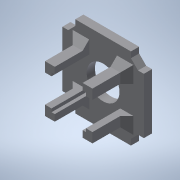
# Autodesk Inventor part: 20_Cube_Insert_Beamsplitter_v3
Saved by Autodesk Inventor 2022 (Build 260153000, 153)
## iProperties
Created: 2019-08-06
Part Number: 20_Cube_Insert_Beamsplitter_v3
Material: Generic
Document SubType Name: Modeling
Designer: marsikovabarbora
Density: 1 g/cm^3
Appearance: Default
Author: marsikovabarbora
Autodesk Inventor part; units mm, degrees
ref_plane "YZ Plane" through (0, 0, 0) normal (1, 0, 0) x (0, 1, 0)
ref_plane "XZ Plane" through (0, 0, 0) normal (0, 1, 0) x (-1, 0, 0)
ref_plane "XY Plane" through (0, 0, 0) normal (0, 0, 1) x (1, 0, 0)
sketch "Sketch1" plane through (0, 0, 0) normal (0, 0, 1) x (1, 0, 0)
  line L0 (-34.86, 0) -> (34.86, 0) construction
  line L1 (0, -34.86) -> (0, 34.86) construction
  line L2 (0, 0) -> (16.9726, 16.9726) construction
  line L3 (0, 0) -> (24.0028, 0) construction
  line L4 (0, 24.9) -> (16.8009, 24.9)
  line L5 (16.8009, 24.9) -> (16.8009, 21.2415)
  line L6 (16.8009, 21.2415) -> (19.0212, 19.0212)
  line L7 (24.9, 0) -> (24.9, 16.8009)
  line L8 (24.9, 16.8009) -> (21.2415, 16.8009)
  line L9 (21.2415, 16.8009) -> (19.0212, 19.0212)
  line L10 (0, -24.9) -> (16.8009, -24.9)
  line L11 (16.8009, -24.9) -> (16.8009, -21.2415)
  line L12 (16.8009, -21.2415) -> (19.0212, -19.0212)
  line L13 (24.9, 0) -> (24.9, -16.8009)
  line L14 (24.9, -16.8009) -> (21.2415, -16.8009)
  line L15 (21.2415, -16.8009) -> (19.0212, -19.0212)
  line L16 (0, 0) -> (-16.9726, 16.9726) construction
  line L17 (0, 0) -> (-24.0028, 0) construction
  line L18 (0, 24.9) -> (-16.8009, 24.9)
  line L19 (-16.8009, 24.9) -> (-16.8009, 21.2415)
  line L20 (-16.8009, 21.2415) -> (-19.0212, 19.0212)
  line L21 (-24.9, 0) -> (-24.9, 16.8009)
  line L22 (-24.9, 16.8009) -> (-21.2415, 16.8009)
  line L23 (-21.2415, 16.8009) -> (-19.0212, 19.0212)
  line L24 (0, -24.9) -> (-16.8009, -24.9)
  line L25 (-16.8009, -24.9) -> (-16.8009, -21.2415)
  line L26 (-16.8009, -21.2415) -> (-19.0212, -19.0212)
  line L27 (-21.2415, -16.8009) -> (-19.0212, -19.0212)
  line L28 (-24.9, -16.8009) -> (-21.2415, -16.8009)
  line L29 (-24.9, 0) -> (-24.9, -16.8009)
  circle A0 centre (0, 0) radius 10
  dimension "d17" = 45
  dimension "d18" = 24.9
  dimension "d20" = 3.14
  dimension "d21" = 26.9
  dimension "d22" = 20
  constraints: 56 end point, 22 symmetric about line, 3 point on line, 2 horizontal, 2 perpendicular, 1 centre point, 1 coincident, 1 equal length
  measures "d17" angle of L3 L2
  measures "d18" distance between parallel lines of L0 L4
  measures "d20" distance of L5.end L6.end
  measures "d21" distance from line of L2.start L6
  measures "d22" diameter of A0
extrude "Extrusion1" add sketch "Sketch1" along normal blind 5
sketch "Skizze6" plane through (0, 0, 5) normal (0, 0, 1) x (1, 0, 0)
  circle A0 centre (0, 0) radius 10 construction
  line L0 (16.8009, 24.9) -> (-16.8009, 24.9) construction
  line L1 (-16.8009, 24.9) -> (-16.8009, 21.2415) projected
  line L2 (-16.8009, 21.2415) -> (-21.2415, 16.8009) projected
  line L3 (-21.2415, 16.8009) -> (-24.9, 16.8009) projected
  line L4 (-24.9, 16.8009) -> (-24.9, -16.8009) construction
  line L5 (-24.9, -16.8009) -> (-21.2415, -16.8009) projected
  line L6 (-21.2415, -16.8009) -> (-16.8009, -21.2415) projected
  line L7 (-16.8009, -21.2415) -> (-16.8009, -24.9) projected
  line L8 (-16.8009, -24.9) -> (16.8009, -24.9) construction
  line L9 (16.8009, -24.9) -> (16.8009, -21.2415) projected
  line L10 (16.8009, -21.2415) -> (21.2415, -16.8009) projected
  line L11 (21.2415, -16.8009) -> (24.9, -16.8009) projected
  line L12 (24.9, -16.8009) -> (24.9, 16.8009) construction
  line L13 (24.9, 16.8009) -> (21.2415, 16.8009) projected
  line L14 (21.2415, 16.8009) -> (16.8009, 21.2415) projected
  line L15 (16.8009, 21.2415) -> (16.8009, 24.9) projected
  line L16 (-17.0009, 25.1) -> (17.0009, 25.1) construction
  line L17 (17.0009, 25.1) -> (17.0009, 21.3243)
  line L18 (17.0009, 21.3243) -> (21.3243, 17.0009)
  line L19 (21.3243, 17.0009) -> (25.1, 17.0009)
  line L20 (25.1, 17.0009) -> (25.1, -17.0009) construction
  line L21 (25.1, -17.0009) -> (21.3243, -17.0009)
  line L22 (21.3243, -17.0009) -> (17.0009, -21.3243)
  line L23 (17.0009, -21.3243) -> (17.0009, -25.1)
  line L24 (17.0009, -25.1) -> (-17.0009, -25.1) construction
  line L25 (-17.0009, -25.1) -> (-17.0009, -21.3243)
  line L26 (-17.0009, -21.3243) -> (-21.3243, -17.0009)
  line L27 (-21.3243, -17.0009) -> (-25.1, -17.0009)
  line L28 (-25.1, -17.0009) -> (-25.1, 17.0009) construction
  line L29 (-25.1, 17.0009) -> (-21.3243, 17.0009)
  line L30 (-21.3243, 17.0009) -> (-17.0009, 21.3243)
  line L31 (-17.0009, 21.3243) -> (-17.0009, 25.1)
  line L32 (-24.9, 16.8009) -> (-24.9, 17.0009)
  line L33 (-16.8009, 24.9) -> (-17.0009, 24.9)
  line L34 (16.8009, 24.9) -> (-16.8009, 24.9) projected
  line L35 (16.8009, 24.9) -> (17.0009, 24.9)
  line L36 (24.9, 16.8009) -> (24.9, 17.0009)
  line L37 (16.8009, -24.9) -> (17.0009, -24.9)
  line L38 (21.2415, -16.8009) -> (24.9, -16.8009) projected
  line L39 (24.9, -16.8009) -> (24.9, -17.0009)
  line L40 (-16.8009, -24.9) -> (-17.0009, -24.9)
  line L41 (-24.9, -16.8009) -> (-21.2415, -16.8009) projected
  line L42 (-24.9, -16.8009) -> (-24.9, -17.0009)
  dimension "d17" = 45
  dimension "d18" = 24.9
  dimension "d20" = 3.14
  dimension "d21" = 26.9
  dimension "d41" = 0.2
  constraints: 48 end point, 12 point on line, 3 perpendicular, 1 vertical, 15 other
  measures "d41" distance between parallel lines of L0 L16
extrude "IM_offset" add sketch "Skizze6" against normal up to surface (5 mm away)
sketch "Sketch8" plane through (0, 0, 5) normal (0, 0, 1) x (1, 0, 0)
  circle A0 centre (0, 0) radius 10 projected
  line L0 (-10.5, -10.5) -> (10.5, -10.5)
  line L1 (10.5, -10.5) -> (10.5, 10.5)
  line L2 (10.5, 10.5) -> (-10.5, 10.5)
  line L3 (-10.5, 10.5) -> (-10.5, -10.5)
  line L4 (-10.5, -10.5) -> (10.5, 10.5) construction
  line L5 (10.5, -10.5) -> (-10.5, 10.5) construction
  line L6 (-10.5, -10.5) -> (10.5, -10.5) construction
  line L7 (14.5, 14.5) -> (14.5, -14.5)
  line L8 (14.5, -14.5) -> (-14.5, -14.5)
  line L9 (-14.5, -14.5) -> (-14.5, 14.5)
  line L10 (-14.5, 14.5) -> (14.5, 14.5)
  dimension "d48" = 21
  dimension "d49" = 0
  dimension "d50" = 21
  dimension "d51" = 4
  constraints: 22 end point, 4 parallel, 2 midpoint, 2 perpendicular, 1 collinear, 1 horizontal, 3 other
  measures "d48" distance of L0.start L0.end
  measures "d49" distance between parallel lines of L6 L0
  measures "d50" distance of L1.end L0.end
  measures "d51" distance between parallel lines of L1 L7
extrude "Extrusion8" add sketch "Sketch8" along normal blind 21 contours L7 L8 L9 L10
sketch "Sketch9" plane through (0, 0, 26) normal (0, 0, 1) x (1, 0, 0)
  line L0 (17.0009, 24.9) -> (-17.0009, 24.9) projected
  line L1 (-17.0009, 24.9) -> (-17.0009, 21.3243) projected
  line L2 (-17.0009, 21.3243) -> (-21.3243, 17.0009) projected
  line L3 (-21.3243, 17.0009) -> (-24.9, 17.0009) projected
  line L4 (-24.9, 17.0009) -> (-24.9, -17.0009) projected
  line L5 (-24.9, -17.0009) -> (-21.3243, -17.0009) projected
  line L6 (-21.3243, -17.0009) -> (-17.0009, -21.3243) projected
  line L7 (-17.0009, -21.3243) -> (-17.0009, -24.9) projected
  line L8 (-17.0009, -24.9) -> (17.0009, -24.9) projected
  line L9 (17.0009, -24.9) -> (17.0009, -21.3243) projected
  line L10 (17.0009, -21.3243) -> (21.3243, -17.0009) projected
  line L11 (21.3243, -17.0009) -> (24.9, -17.0009) projected
  line L12 (24.9, -17.0009) -> (24.9, 17.0009) projected
  line L13 (24.9, 17.0009) -> (21.3243, 17.0009) projected
  line L14 (21.3243, 17.0009) -> (17.0009, 21.3243) projected
  line L15 (17.0009, 21.3243) -> (17.0009, 24.9) projected
  line L16 (-14.5, 14.5) -> (14.5, 14.5) projected
  line L17 (14.5, 14.5) -> (14.5, -14.5) projected
  line L18 (14.5, -14.5) -> (-14.5, -14.5) projected
  line L19 (-14.5, -14.5) -> (-14.5, 14.5) projected
  line L20 (24.9, -8.5) -> (-24.9, -8.5)
  line L21 (-24.9, -8.5) -> (-24.9, 8.5)
  line L22 (-24.9, 8.5) -> (24.9, 8.5)
  line L23 (24.9, 8.5) -> (24.9, -8.5)
  line L24 (24.9, -8.5) -> (-24.9, 8.5) construction
  line L25 (-24.9, -8.5) -> (24.9, 8.5) construction
  line L26 (8.5, -24.9) -> (8.5, 24.9)
  line L27 (8.5, 24.9) -> (-8.5, 24.9)
  line L28 (-8.5, 24.9) -> (-8.5, -24.9)
  line L29 (-8.5, -24.9) -> (8.5, -24.9)
  line L30 (8.5, -24.9) -> (-8.5, 24.9) construction
  line L31 (8.5, 24.9) -> (-8.5, -24.9) construction
  point P0 (0, 0)
  point P1 (-8.5, -8.5)
  point P2 (8.5, -8.5)
  point P3 (8.5, 8.5)
  point P4 (-8.5, 8.5)
  dimension "d54" = 17
  dimension "d55" = 17
  constraints: 24 end point, 4 midpoint, 4 parallel, 2 perpendicular
  measures "d54" distance of L20.end L21.end
  measures "d55" distance of L27.end L26.end
extrude "Extrusion9" cut sketch "Sketch9" against normal blind 21 contours L26 L16 L28 L0 | L26 L22 L28 L16 | L26 L20 L28 L22 | L22 L17 L20 L26 | L28 L20 L19 L22 | L22 L12 L20 L17 | L26 L18 L28 L20 | L19 L20 L4 L22 | L26 L8 L28 L18
chamfer "Chamfer1" distance 4 angle 45 8 edges at (-11.5, 14.5, 5) (11.5, 14.5, 5) (-14.5, 11.5, 5) (-14.5, -11.5, 5) (-11.5, -14.5, 5) (11.5, -14.5, 5) (14.5, -11.5, 5) (14.5, 11.5, 5)
body "Solid1"
